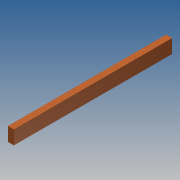
# Autodesk Inventor part: hubjig_side1
Saved by Autodesk Inventor 2014 SP1 (Build 180222100, 222)
## iProperties
Created: 2014-08-29
Part Number: hubjig_side1
Material: Wood (Cherry)
Document SubType Name: Modeling
Designer: Dave
Mass: 2168.01 g
Surface Area: 2648.38 cm^2
Volume: 3441.28 cm^3
Density: 0.63 g/cm^3
Appearance: Cherry - Natural Low Gloss
Author: Dave
Autodesk Inventor part; units mm, degrees
ref_plane "YZ Plane" through (0, 0, 0) normal (1, 0, 0) x (0, 1, 0)
ref_plane "XZ Plane" through (0, 0, 0) normal (0, 1, 0) x (-1, 0, 0)
ref_plane "XY Plane" through (0, 0, 0) normal (0, 0, 1) x (1, 0, 0)
sketch "Sketch1" plane through (0, 0, 0) normal (0, 0, 1) x (1, 0, 0)
  line L0 (0, 0) -> (38.1, 0)
  line L1 (38.1, 0) -> (38.1, 88.9)
  line L2 (38.1, 88.9) -> (0, 88.9)
  line L3 (0, 88.9) -> (0, 0)
  dimension "d0" = 38.1
  dimension "d1" = 88.9
  constraints: 8 end point, 2 parallel, 1 horizontal, 1 perpendicular
  measures "d0" distance of L0.start L0.end
  measures "d1" distance of L2.end L0.start
extrude "Extrusion1" add sketch "Sketch1" along normal blind 1016
sketch "Sketch2" plane through (38.1, 0, 0) normal (1, 0, 0) x (0, 0, -1)
  line L0 (-1016, 0) -> (-1016, 88.9) projected
  line L1 (0, 0) -> (-1016, 0) projected
  circle A0 centre (-996.95, 19.05) radius 9.6959
  circle A1 centre (-19.05, 19.05) radius 9.6959
  circle A2 centre (-996.95, 69.85) radius 9.6959
  circle A3 centre (-19.05, 69.85) radius 9.6959
  dimension "d4" = 19.05
  dimension "d5" = 19.05
  dimension "d8" = 977.9
  dimension "d11" = 50.8
  constraints: 4 centre point, 1 horizontal, 1 vertical, 6 other
  measures "d4" distance from line of A0.centre L1
  measures "d5" distance from line of L0 A0.centre
  measures "d8" distance of A0.centre A1.centre
  measures "d11" distance of A0.centre A2.centre
hole "Hole1" at (38.1, 69.85, 996.95) at (38.1, 19.05, 996.95) at (38.1, 69.85, 19.05) at (38.1, 19.05, 19.05) direction (-1, 0, 0) diameter 5.1054 end through all clearance for "Flat Head Machine Screw (82)" size "#10" standard "Ansi Unified Screw Threads"
body "Solid1"
